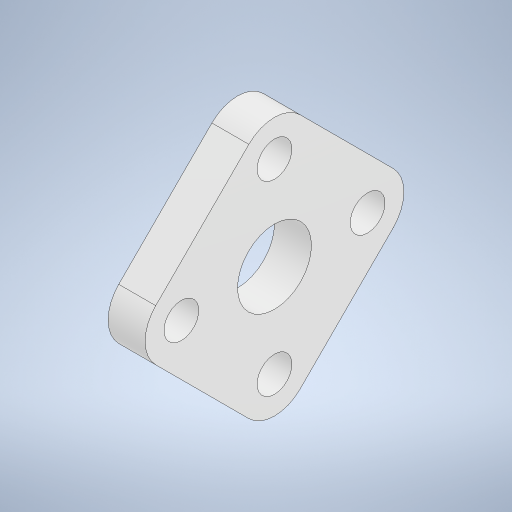
# Autodesk Inventor part: Brace
Saved by Autodesk Inventor 2023.2 (Build 272271000, 271)
## iProperties
Created: 2023-06-28
Part Number: Brace
Material: UHMW, White
Document SubType Name: Modeling
Designer: Nathan Cai
Density: 0.94 g/cm^3
Appearance: Smooth - White
Mass: 0.618982 g
Surface Area: 8.30039 cm^2
Volume: 0.658491 cm^3
Author: Nathan Cai
Autodesk Inventor part; units mm, degrees
ref_plane "YZ Plane" through (0, 0, 0) normal (1, 0, 0) x (0, 1, 0)
ref_plane "XZ Plane" through (0, 0, 0) normal (0, 1, 0) x (-1, 0, 0)
ref_plane "XY Plane" through (0, 0, 0) normal (0, 0, 1) x (1, 0, 0)
sketch "Sketch1" plane through (0, 0, 0) normal (1, 0, 0) x (0, 1, 0)
  circle A0 centre (0, 0) radius 11.1125
  line L0 (0, 0) -> (11.1125, 0)
  circle A1 centre (0, 0) radius 8 construction
  circle A2 centre (8, 0) radius 1.5
  circle A3 centre (5.6569, 5.6569) radius 1.5
  circle A4 centre (0, 8) radius 1.5
  circle A5 centre (-5.6569, 5.6569) radius 1.5
  circle A6 centre (-8, 0) radius 1.5
  circle A7 centre (-5.6569, -5.6569) radius 1.5
  circle A8 centre (0, -8) radius 1.5
  circle A9 centre (5.6569, -5.6569) radius 1.5
  circle A10 centre (0, 0) radius 3.175
  line L1 (-12.4017, 0) -> (0, 12.4017)
  line L2 (0, 12.4017) -> (12.4017, 0)
  line L3 (12.4017, 0) -> (0, -12.4017)
  line L4 (0, -12.4017) -> (-12.4017, 0)
  circle A11 centre (0, 8) radius 3.1125
  circle A12 centre (-8, 0) radius 3.1125
  circle A13 centre (0, -8) radius 3.1125
  circle A14 centre (8, 0) radius 3.1125
  point P0 (10.2009, 2.2009)
  point P1 (2.2009, 10.2009)
  point P2 (-2.2009, 10.2009)
  point P3 (-10.2009, 2.2009)
  point P4 (-10.2009, -2.2009)
  point P5 (-2.2009, -10.2009)
  point P6 (2.2009, -10.2009)
  point P7 (10.2009, -2.2009)
  dimension "d0" = 22.225
  dimension "d1" = 16
  dimension "d2" = 3
  dimension "d5" = 360
  dimension "d7" = 6.35
  dimension "d12" = 360
  constraints: 13 centre point, 10 end point, 5 coincident, 2 horizontal alignment, 2 tangent, 1 horizontal, 1 point on line, 40 other
  measures "d2" diameter of A2
  measures "d7" diameter of A10
extrude "Extrusion1" add sketch "Sketch1" along normal blind 3.175 contours A14 L0 A2 | L0 A2 A14 | A14 L3 A9 A13 L4 A7 A12 L1 A5 A11 L2 A3 | A3 L2 | L3 A9 | A11 | A13 | A5 L1 | L4 A7 | A12 picked at (5.5263, 5.9374) picked at (5.3691, -6.0323) picked at (-5.9998, 5.4528) picked at (-5.3149, -5.4172)
body "Solid1"
